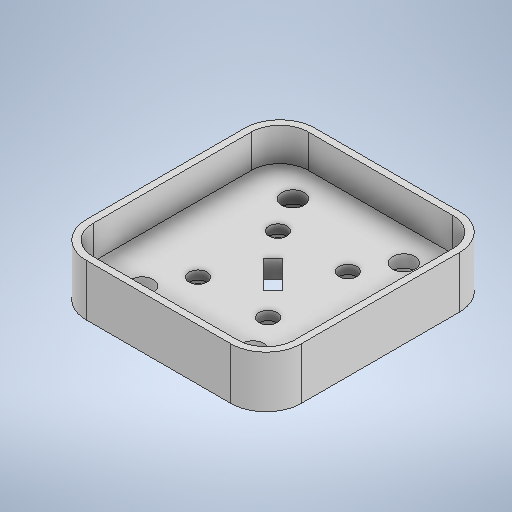
# Autodesk Inventor part: Pin-Cradle
Saved by Autodesk Inventor 2025 (Build 290162000, 162)
## iProperties
Created: 2025-03-04
Part Number: Pin-Cradle
Material: Generic
Document SubType Name: Modeling
Designer: maxsm
Density: 1 g/cm^3
Appearance: Default
Author: maxsm
Autodesk Inventor part; units mm, degrees
ref_plane "YZ Plane" through (0, 0, 0) normal (1, 0, 0) x (0, 1, 0)
ref_plane "XZ Plane" through (0, 0, 0) normal (0, 1, 0) x (-1, 0, 0)
ref_plane "XY Plane" through (0, 0, 0) normal (0, 0, 1) x (1, 0, 0)
sketch "Sketch1" plane through (0, 0, 0) normal (0, 1, 0) x (-1, 0, 0)
  line L0 (16.25, 25.8) -> (-16.25, 25.8)
  line L1 (-24.25, 17.8) -> (-24.25, -17.8)
  line L2 (-16.25, -25.8) -> (16.25, -25.8)
  line L3 (24.25, -17.8) -> (24.25, 17.8)
  line L4 (24.25, 25.8) -> (-24.25, -25.8) construction
  line L5 (-24.25, 25.8) -> (24.25, -25.8) construction
  arc A0 (24.25, 17.8) -> (16.25, 25.8) centre (16.25, 17.8) ccw
  arc A1 (16.25, -25.8) -> (24.25, -17.8) centre (16.25, -17.8) ccw
  arc A2 (-24.25, -17.8) -> (-16.25, -25.8) centre (-16.25, -17.8) ccw
  arc A3 (-16.25, 25.8) -> (-24.25, 17.8) centre (-16.25, 17.8) ccw
  point P0 (0, 0)
  dimension "d1" = 48.5
  dimension "d2" = 51.6
  dimension "d3" = 8
  constraints: 12 end point, 8 point on circle, 8 point on line, 8 tangent, 4 centre point, 3 equal radius, 2 midpoint, 2 parallel, 1 horizontal, 1 perpendicular
  measures "d1" distance between parallel lines of L1 L3
  measures "d2" distance between parallel lines of L0 L2
  measures "d3" radius of A0
extrude "Extrusion1" add sketch "Sketch1" along normal blind 9
shell "Shell1" thickness 1.5 removed faces 1 at (8.0833, 9, -5.9333)
thicken "Thicken1" operation add thickness 2.65 both sides no extend neighbours no toward (0, -1, 0) faces at (8.0833, 0, -5.9333)
sketch "Sketch2" plane through (-16.25, 1.5, -24.3) normal (0, 1, 0) x (1, 0, 0)
  line L0 (18.3713, -28.5426) -> (12.0074, -22.1787)
  line L1 (12.0074, -22.1787) -> (14.1287, -20.0574)
  line L2 (14.1287, -20.0574) -> (20.4926, -26.4213)
  line L3 (20.4926, -26.4213) -> (18.3713, -28.5426)
  line L4 (18.3713, -28.5426) -> (14.1287, -20.0574) construction
  line L5 (12.0074, -22.1787) -> (20.4926, -26.4213) construction
  line L6 (18.3713, -28.5426) -> (27.3713, -28.5426) construction
  line L7 (-6.5, -42.1) -> (-6.5, -6.5) construction
  line L8 (0, 0) -> (32.5, 0) construction
  circle A0 centre (8.35, -15.3) radius 1.05
  circle A1 centre (8.35, -33.3) radius 1.05
  line L9 (-17.7, -24.3) -> (50.2, -24.3) projected
  circle A2 centre (24.15, -15.3) radius 1.05
  circle A3 centre (24.15, -33.3) radius 1.05
  line L10 (16.25, 11.82) -> (16.25, -60.42) projected
  point P0 (16.25, -24.3)
  point P1 (16.25, -24.3)
  point P2 (16.25, -24.3)
  dimension "d12" = 9
  dimension "d13" = 135
  dimension "d14" = 3
  dimension "d15" = 22.75
  dimension "d16" = 24.3
  dimension "d19" = 7.9
  dimension "d20" = 2.1
  dimension "d21" = 18
  constraints: 14 end point, 4 centre point, 4 midpoint, 3 equal radius, 2 parallel, 2 symmetric about line, 2 vertical alignment, 1 equal length, 1 horizontal, 1 horizontal alignment, 1 perpendicular
  measures "d12" distance of L0.start L0.end
  measures "d13" angle of L6 L0
  measures "d14" distance of L0.end L1.end
  measures "d15" distance from line of point (16.25, -24.3) L7
  measures "d16" distance from line of point (16.25, -24.3) L8
  measures "d19" horizontal distance of point (16.25, -24.3) A0.centre
  measures "d20" diameter of A0
  measures "d21" distance of A1.centre A0.centre
extrude "Extrusion2" cut sketch "Sketch2" against normal through all
sketch "Sketch3" plane through (-16.25, 1.5, -24.3) normal (0, 1, 0) x (1, 0, 0)
  circle A0 centre (3.75, -7.3) radius 2.5
  circle A1 centre (28.75, -7.3) radius 2.5
  circle A2 centre (3.75, -41.3) radius 2.5
  circle A3 centre (28.75, -41.3) radius 2.5
  point P0 (16.25, -24.3)
  dimension "d22" = 5
  dimension "d23" = 25
  dimension "d24" = 34
  dimension "d25" = 17
  dimension "d26" = 12.5
  constraints: 4 centre point, 3 equal radius, 2 horizontal alignment, 2 vertical alignment
  measures "d22" diameter of A0
  measures "d23" distance of A1.centre A0.centre
  measures "d24" distance of A2.centre A0.centre
  measures "d25" vertical distance of A0.centre point (16.25, -24.3)
  measures "d26" horizontal distance of point (16.25, -24.3) A0.centre
extrude "Extrusion3" cut sketch "Sketch3" against normal blind 2.8
sketch "Sketch4" plane through (-16.25, 1.5, -24.3) normal (0, 1, 0) x (1, 0, 0)
  circle A0 centre (8.35, -15.3) radius 2
  circle A1 centre (8.35, -33.3) radius 1.05 projected
  circle A2 centre (8.35, -33.3) radius 2
  circle A3 centre (8.35, -15.3) radius 1.05 projected
  circle A4 centre (24.15, -15.3) radius 2
  circle A5 centre (24.15, -33.3) radius 2
  circle A6 centre (24.15, -15.3) radius 1.05 projected
  circle A7 centre (24.15, -33.3) radius 1.05 projected
  point P0 (16.25, -24.3)
  dimension "d29" = 4
  constraints: 4 centre point, 3 concentric, 3 equal radius, 1 coincident
  measures "d29" diameter of A0
extrude "Extrusion4" cut sketch "Sketch4" against normal blind 2
sketch "Sketch5" plane through (-16.25, -2.65, 25.8) normal (0, -1, 0) x (1, 0, 0)
  line L0 (-8, -43.6) -> (-8, -8) projected
  line L1 (-8, -39.8) -> (-15.65, -39.8)
  line L2 (-15.65, -39.8) -> (-15.65, -11.8)
  line L3 (-15.65, -11.8) -> (-8, -11.8)
  line L4 (-8, -11.8) -> (-8, -39.8)
  line L5 (-24.48, -25.8) -> (51.33, -25.8) projected
  line L6 (-15.65, -39.8) -> (-8, -39.8)
  line L7 (-8, -39.8) -> (-8, -30.8)
  line L8 (-8, -30.8) -> (-15.65, -30.8)
  line L9 (-15.65, -30.8) -> (-15.65, -39.8)
  circle A0 centre (-10.65, -34.8) radius 1.05
  point P0 (16.25, -25.8)
  point P1 (-8, -11.8)
  point P2 (-8, -30.8)
  point P3 (-15.65, -30.8)
  dimension "d34" = 7.65
  dimension "d35" = 28
  dimension "d37" = 9
  dimension "d38" = 5
  dimension "d39" = 5
  dimension "d40" = 2.1
  constraints: 16 end point, 4 parallel, 2 horizontal, 2 perpendicular, 2 point on line, 1 centre point, 1 other
  measures "d34" distance between parallel lines of L0 L2
  measures "d35" distance between parallel lines of L3 L1
  measures "d37" distance between parallel lines of L1 L8
  measures "d38" distance from line of A0.centre L1
  measures "d39" distance from line of A0.centre L2
  measures "d40" diameter of A0
extrude "Extrusion5" add sketch "Sketch5" against normal blind 2.15 contours L1 L2 L8 L0
fillet "Fillet1" radius 3 1 edges at (-31.9, -1.575, -14)
mirror "Mirror1" about plane through (0, 0, 0) normal (0, 0, 1) of "Extrusion5", "Fillet1"
equation "\"d25\" = 0.5 * d24"
equation "\"d26\" = 0.5 * d23"
body "Solid1"
